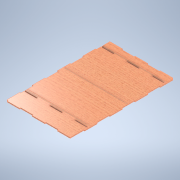
# Autodesk Inventor part: Wall_V1
Saved by Autodesk Inventor 2022.2 (Build 262287000, 287)
## iProperties
Created: 2022-11-15
Part Number: Wall_V1
Material: Generic
Document SubType Name: Modeling
Designer: jaege
Density: 1 g/cm^3
Appearance: Red Oak - Natural Low Gloss
Author: jaege
Autodesk Inventor part; units mm, degrees
ref_plane "YZ Plane" through (0, 0, 0) normal (1, 0, 0) x (0, 1, 0)
ref_plane "XZ Plane" through (0, 0, 0) normal (0, 1, 0) x (-1, 0, 0)
ref_plane "XY Plane" through (0, 0, 0) normal (0, 0, 1) x (1, 0, 0)
sketch "Sketch1" plane through (0, 0, 0) normal (0, 1, 0) x (-1, 0, 0)
  line L0 (-125, 200) -> (125, 200) construction
  line L1 (125, 200) -> (125, -200) construction
  line L2 (125, -200) -> (-125, -200) construction
  line L3 (-125, -200) -> (-125, 200) construction
  line L4 (-125, 200) -> (125, -200) construction
  line L5 (125, 200) -> (-125, -200) construction
  line L6 (125, 200) -> (75, 200) construction
  line L7 (75, 200) -> (75, 204)
  line L8 (75, 204) -> (125, 204)
  line L9 (125, 204) -> (125, 200)
  line L10 (125, 200) -> (129, 200)
  line L11 (129, 200) -> (129, 150)
  line L12 (129, 150) -> (125, 150)
  line L13 (125, 150) -> (125, 200) construction
  line L14 (-125, 200) -> (-129, 200) construction
  line L15 (-129, 200) -> (-129, 150) construction
  line L16 (-129, 150) -> (-125, 150)
  line L17 (-125, 150) -> (-125, 200)
  line L18 (125, -200) -> (75, -200) construction
  line L19 (75, -200) -> (75, -204)
  line L20 (75, -204) -> (125, -204)
  line L21 (125, -204) -> (125, -200)
  line L22 (125, 100) -> (125, 150)
  line L23 (125, 150) -> (129, 150)
  line L24 (129, 100) -> (125, 100)
  line L25 (129, 150) -> (129, 100) construction
  line L26 (-125, 100) -> (-125, 150) construction
  line L27 (-125, 150) -> (-129, 150)
  line L28 (-129, 150) -> (-129, 100)
  line L29 (-129, 100) -> (-125, 100)
  line L30 (125, 50) -> (125, 100) construction
  line L31 (125, 100) -> (129, 100)
  line L32 (129, 50) -> (125, 50)
  line L33 (129, 100) -> (129, 50)
  line L34 (-125, 50) -> (-125, 100)
  line L35 (-125, 100) -> (-129, 100)
  line L36 (-129, 100) -> (-129, 50) construction
  line L37 (-129, 50) -> (-125, 50)
  line L38 (125, 0) -> (125, 50)
  line L39 (125, 50) -> (129, 50)
  line L40 (129, 0) -> (125, 0)
  line L41 (129, 50) -> (129, 0) construction
  line L42 (-125, 0) -> (-125, 50) construction
  line L43 (-125, 50) -> (-129, 50)
  line L44 (-129, 50) -> (-129, 0)
  line L45 (-129, 0) -> (-125, 0)
  line L46 (125, -50) -> (125, 0) construction
  line L47 (125, 0) -> (129, 0)
  line L48 (129, -50) -> (125, -50)
  line L49 (129, 0) -> (129, -50)
  line L50 (-125, -50) -> (-125, 0)
  line L51 (-125, 0) -> (-129, 0)
  line L52 (-129, 0) -> (-129, -50) construction
  line L53 (-129, -50) -> (-125, -50)
  line L54 (125, -100) -> (125, -50)
  line L55 (125, -50) -> (129, -50)
  line L56 (129, -100) -> (125, -100)
  line L57 (129, -50) -> (129, -100) construction
  line L58 (-125, -100) -> (-125, -50) construction
  line L59 (-125, -50) -> (-129, -50)
  line L60 (-129, -50) -> (-129, -100)
  line L61 (-129, -100) -> (-125, -100)
  line L62 (125, -150) -> (125, -100) construction
  line L63 (125, -100) -> (129, -100)
  line L64 (129, -150) -> (125, -150)
  line L65 (129, -100) -> (129, -150)
  line L66 (-125, -150) -> (-125, -100)
  line L67 (-125, -100) -> (-129, -100)
  line L68 (-129, -100) -> (-129, -150) construction
  line L69 (-129, -150) -> (-125, -150)
  line L70 (125, -200) -> (125, -150)
  line L71 (125, -150) -> (129, -150)
  line L72 (129, -200) -> (125, -200) construction
  line L73 (129, -150) -> (129, -200) construction
  line L74 (-125, -200) -> (-125, -150) construction
  line L75 (-125, -150) -> (-129, -150)
  line L76 (-129, -150) -> (-129, -200)
  line L77 (-129, -200) -> (-125, -200)
  line L78 (75, 204) -> (75, 200)
  line L79 (25, 200) -> (25, 204)
  line L80 (25, 204) -> (75, 204) construction
  line L81 (75, 200) -> (25, 200)
  line L82 (75, -200) -> (25, -200)
  line L83 (25, -200) -> (25, -204)
  line L84 (25, -204) -> (75, -204) construction
  line L85 (75, -204) -> (75, -200)
  line L86 (25, 204) -> (25, 200)
  line L87 (-25, 200) -> (-25, 204)
  line L88 (-25, 204) -> (25, 204)
  line L89 (25, 200) -> (-25, 200) construction
  line L90 (25, -200) -> (-25, -200) construction
  line L91 (-25, -200) -> (-25, -204)
  line L92 (-25, -204) -> (25, -204)
  line L93 (25, -204) -> (25, -200)
  line L94 (-25, 204) -> (-25, 200)
  line L95 (-75, 200) -> (-75, 204)
  line L96 (-75, 204) -> (-25, 204) construction
  line L97 (-25, 200) -> (-75, 200)
  line L98 (-25, -200) -> (-75, -200)
  line L99 (-75, -200) -> (-75, -204)
  line L100 (-75, -204) -> (-25, -204) construction
  line L101 (-25, -204) -> (-25, -200)
  line L102 (-75, 204) -> (-75, 200)
  line L103 (-125, 200) -> (-125, 204)
  line L104 (-125, 204) -> (-75, 204)
  line L105 (-75, 200) -> (-125, 200) construction
  line L106 (-75, -200) -> (-125, -200) construction
  line L107 (-125, -200) -> (-125, -204)
  line L108 (-125, -204) -> (-75, -204)
  line L109 (-75, -204) -> (-75, -200)
  point P0 (0, 0)
  dimension "d0" = 250
  dimension "d1" = 400
  dimension "d2" = 50
  dimension "d3" = 4
  dimension "d4" = 4
  dimension "d5" = 50
  dimension "d6" = 4
  dimension "d7" = 50
  dimension "d8" = 50
  dimension "d9" = 4
  dimension "d12" = 50
  dimension "d19" = 50
  constraints: 220 end point, 10 parallel, 6 horizontal, 5 perpendicular, 2 midpoint, 1 vertical, 180 other
  measures "d0" distance of L1.end L2.end
  measures "d1" distance of L0.end L1.end
  measures "d2" distance of L7.end L8.end
  measures "d3" distance of L6.end L7.end
  measures "d4" distance of L11.end L12.end
  measures "d5" distance of L10.end L11.end
  measures "d6" distance of L16.end L15.end
  measures "d7" distance of L15.end L14.end
  measures "d8" distance of L20.end L19.end
  measures "d9" distance of L19.end L18.end
  measures "d12" distance of L0.end L22.end
  measures "d19" distance of L0.end L78.end
extrude "Extrusion1" add sketch "Sketch1" along normal blind 4
sketch "Sketch3" plane through (0, 4, 0) normal (0, 1, 0) x (1, 0, 0)
  line L0 (-129, 50) -> (-129, 0) projected
  line L1 (-129, 25) -> (125, 25) construction
  line L2 (125, 0) -> (125, 50) projected
  line L3 (-129, 22.5) -> (125, 22.5)
  line L4 (125, 22.5) -> (125, 27.5)
  line L5 (125, 27.5) -> (-129, 27.5)
  line L6 (-129, 27.5) -> (-129, 22.5)
  line L7 (-129, 27.5) -> (-125, 27.5)
  line L8 (-125, 27.5) -> (-125, 22.5)
  line L9 (-125, 22.5) -> (-129, 22.5)
  line L10 (-129, 22.5) -> (-129, 27.5)
  line L11 (-25, -200) -> (-25, -204) projected
  line L12 (-25, -204) -> (25, -204) projected
  line L13 (25, -204) -> (25, -200) projected
  line L14 (25, -200) -> (75, -200) projected
  line L15 (75, -200) -> (75, -204) projected
  line L16 (75, -204) -> (125, -204) projected
  line L17 (125, -204) -> (125, -150) projected
  line L18 (125, -150) -> (129, -150) projected
  line L19 (129, -150) -> (129, -100) projected
  line L20 (129, -100) -> (125, -100) projected
  line L21 (125, -100) -> (125, -50) projected
  line L22 (125, -50) -> (129, -50) projected
  line L23 (129, -50) -> (129, 0) projected
  line L24 (129, 0) -> (125, 0) projected
  line L25 (125, 0) -> (125, 50) projected
  line L26 (125, 50) -> (129, 50) projected
  line L27 (129, 50) -> (129, 100) projected
  line L28 (129, 100) -> (125, 100) projected
  line L29 (125, 100) -> (125, 150) projected
  line L30 (125, 150) -> (129, 150) projected
  line L31 (129, 150) -> (129, 200) projected
  line L32 (129, 200) -> (125, 200) projected
  line L33 (125, 200) -> (125, 204) projected
  line L34 (125, 204) -> (75, 204) projected
  line L35 (75, 204) -> (75, 200) projected
  line L36 (75, 200) -> (25, 200) projected
  line L37 (25, 200) -> (25, 204) projected
  line L38 (25, 204) -> (-25, 204) projected
  line L39 (-25, 204) -> (-25, 200) projected
  line L40 (-25, 200) -> (-75, 200) projected
  line L41 (-75, 200) -> (-75, 204) projected
  line L42 (-75, 204) -> (-125, 204) projected
  line L43 (-125, 204) -> (-125, 150) projected
  line L44 (-125, 150) -> (-129, 150) projected
  line L45 (-129, 150) -> (-129, 100) projected
  line L46 (-129, 100) -> (-125, 100) projected
  line L47 (-125, 100) -> (-125, 50) projected
  line L48 (-125, 50) -> (-129, 50) projected
  line L49 (-129, 50) -> (-129, 0) projected
  line L50 (-129, 0) -> (-125, 0) projected
  line L51 (-125, 0) -> (-125, -50) projected
  line L52 (-125, -50) -> (-129, -50) projected
  line L53 (-129, -50) -> (-129, -100) projected
  line L54 (-129, -100) -> (-125, -100) projected
  line L55 (-125, -100) -> (-125, -150) projected
  line L56 (-125, -150) -> (-129, -150) projected
  line L57 (-129, -150) -> (-129, -200) projected
  line L58 (-129, -200) -> (-125, -200) projected
  line L59 (-125, -200) -> (-125, -204) projected
  line L60 (-125, -204) -> (-75, -204) projected
  line L61 (-75, -204) -> (-75, -200) projected
  line L62 (-75, -200) -> (-25, -200) projected
  line L63 (-125, -100) -> (-125, -150) projected
  line L64 (-125, -125) -> (129, -125) construction
  line L65 (129, -150) -> (129, -100) projected
  line L66 (-125, -127.5) -> (125, -127.5)
  line L67 (125, -127.5) -> (125, -122.5)
  line L68 (125, -122.5) -> (-125, -122.5)
  line L69 (-125, -122.5) -> (-125, -127.5)
  line L70 (-125, -127.5) -> (125, -122.5) construction
  line L71 (125, -127.5) -> (-125, -122.5) construction
  line L72 (125, 0) -> (125, 50) projected
  line L73 (-125, 0) -> (-125, -50) projected
  line L74 (129, 150) -> (129, 200) projected
  line L75 (129, 175) -> (-125, 175) construction
  line L76 (-125, 172.5) -> (125, 172.5)
  line L77 (125, 172.5) -> (125, 177.5)
  line L78 (125, 177.5) -> (-125, 177.5)
  line L79 (-125, 177.5) -> (-125, 172.5)
  line L80 (-125, 172.5) -> (125, 177.5) construction
  line L81 (125, 172.5) -> (-125, 177.5) construction
  line L82 (-125, 204) -> (-125, 150) projected
  line L83 (125, 100) -> (125, 150) projected
  point P0 (0, 0)
  point P1 (-125, 27.5)
  point P2 (-125, 22.5)
  point P3 (0, -125)
  point P4 (0, 175)
  dimension "d30" = 5
  dimension "d34" = 5
  dimension "d35" = 5
  dimension "d36" = 5
  constraints: 46 end point, 9 midpoint, 8 parallel, 5 collinear, 5 perpendicular, 5 point on line, 4 horizontal, 1 other
  measures "d30" distance of L4.end L3.end
  measures "d34" distance of L7.end L8.end
  measures "d35" distance of L66.end L67.end
  measures "d36" distance of L76.end L77.end
extrude "Extrusion2" cut sketch "Sketch3" against normal blind 1 contours L5 L2 L3 L8 | L43 L78 L77 L76 | L68 L67 L66 L55
sketch "Sketch4" plane through (0, 4, 0) normal (0, 1, 0) x (1, 0, 0)
  line L0 (-125, -133) -> (-75, -133)
  line L1 (-75, -133) -> (-75, -137)
  line L2 (-75, -137) -> (-125, -137)
  line L3 (-125, -137) -> (-125, -133)
  line L4 (-75, -200) -> (-25, -200) projected
  line L5 (125, -127.5) -> (-125, -127.5) projected
  line L6 (-75, -133) -> (-25, -133)
  line L7 (-25, -133) -> (-25, -137)
  line L8 (-25, -137) -> (-75, -137)
  line L9 (-75, -137) -> (-75, -133)
  line L10 (-25, -133) -> (25, -133)
  line L11 (25, -133) -> (25, -137)
  line L12 (25, -137) -> (-25, -137)
  line L13 (-25, -137) -> (-25, -133)
  line L14 (25, -133) -> (75, -133)
  line L15 (75, -133) -> (75, -137)
  line L16 (75, -137) -> (25, -137)
  line L17 (25, -137) -> (25, -133)
  line L18 (75, -133) -> (125, -133)
  line L19 (125, -133) -> (125, -137)
  line L20 (125, -137) -> (75, -137)
  line L21 (75, -137) -> (75, -133)
  line L22 (-125, 0) -> (-125, -50) projected
  line L23 (-125, 172) -> (-75, 172)
  line L24 (-75, 172) -> (-75, 168)
  line L25 (-75, 168) -> (-125, 168)
  line L26 (-125, 168) -> (-125, 172)
  line L27 (-75, 172) -> (-25, 172)
  line L28 (-25, 172) -> (-25, 168)
  line L29 (-25, 168) -> (-25, 172)
  line L30 (-25, 168) -> (-75, 168)
  line L31 (-75, 168) -> (-75, 172)
  line L32 (-25, 172) -> (25, 172)
  line L33 (25, 168) -> (-25, 168)
  line L34 (25, 172) -> (25, 168)
  line L35 (25, 168) -> (25, 172)
  line L36 (25, 172) -> (75, 172)
  line L37 (75, 172) -> (75, 168)
  line L38 (75, 168) -> (75, 172)
  line L39 (75, 172) -> (125, 172)
  line L40 (125, 172) -> (125, 168)
  line L41 (125, 168) -> (75, 168)
  line L42 (75, 168) -> (25, 168)
  point P0 (0, 0)
  point P1 (-125, -135)
  point P2 (-125, -122.5)
  point P3 (-75, -135)
  point P4 (-25, -135)
  point P5 (25, -135)
  point P6 (75, -135)
  point P7 (75, -133)
  point P8 (-25, -133)
  point P9 (-125, 170)
  point P10 (-25, 170)
  point P11 (-75, 170)
  point P12 (25, 170)
  point P13 (75, 170)
  dimension "d37" = 50
  dimension "d38" = 4
  dimension "d39" = 63
  dimension "d42" = 50
  dimension "d51" = 305
  constraints: 80 end point, 2 horizontal, 2 parallel, 1 midpoint, 1 perpendicular, 1 vertical, 1 vertical alignment, 81 other
  measures "d37" distance of L1.end L2.end
  measures "d38" distance of L0.end L1.end
  measures "d39" distance between parallel lines of L4 L2
  measures "d42" distance of L0.start L6.start
  measures "d51" distance of L0.start L23.start
extrude "Extrusion3" cut sketch "Sketch4" against normal up to next contours L0 L1 L2 L3 | L10 L11 L12 L7 | L18 L19 L20 L15 | L23 L24 L25 L26 | L32 L34 L33 L28 | L39 L40 L41 L37
body "Solid1"
